iphone-se3-parametric-drawing-model (Autodesk Fusion 360 design; units mm, degrees)
part number: 2026-09-02-14-29-54-371
part number: 2026-09-02-16-09-22-957
Autodesk Fusion 360 part; units mm, degrees
sketch "スケッチ1" plane through (0, 0, 0) normal (0, 0, 1) x (1, 0, 0) in component "iPhone SE 3 - Parametric Drawing Model"
  arc A0 (33.635, 60.12) -> (24.535, 69.22) centre (24.535, 60.12) ccw
  arc A1 (24.535, -69.22) -> (33.635, -60.12) centre (24.535, -60.12) ccw
  arc A2 (-33.635, -60.12) -> (-24.535, -69.22) centre (-24.535, -60.12) ccw
  arc A3 (-24.535, 69.22) -> (-33.635, 60.12) centre (-24.535, 60.12) ccw
  line L0 (-24.535, 69.22) -> (24.535, 69.22)
  line L1 (33.635, 60.12) -> (33.635, -60.12)
  line L2 (24.535, -69.22) -> (-24.535, -69.22)
  line L3 (-33.635, -60.12) -> (-33.635, 60.12)
  dimension "d710" = 49.07
  dimension "d711" = 120.24
  dimension "d712" = 9.1
  dimension "d713" = 24.535
  dimension "d714" = 60.12
  constraint horizontal L0
  constraint horizontal L2
  constraint vertical L3
  constraint vertical L1
  constraint tangent A0 L0
  constraint tangent A0 L1
  constraint tangent A1 L1
  constraint tangent A1 L2
  constraint tangent A2 L2
  constraint tangent A2 L3
  constraint tangent A3 L3
  constraint tangent A3 L0
  constraint equal A0 A1
  constraint equal A0 A2
  constraint equal A0 A3
  measures "d710" horizontal distance of A0.end A3.start
  measures "d711" vertical distance of A0.start A1.end
  measures "d712" radius of A0
  measures "d713" horizontal distance of origin A0.centre
  measures "d714" vertical distance of origin A0.centre
extrude "Rear Glass" add sketch "スケッチ1" along normal blind 0.9 makes body 1 in component "iPhone SE 3 - Parametric Drawing Model"
ref_plane "作業平面1" through (0, 0, 0.9) normal (0, 0, 1) x (1, 0, 0) in component "iPhone SE 3 - Parametric Drawing Model"
sketch "スケッチ2" plane through (0, 0, 0.9) normal (0, 0, 1) x (1, 0, 0) in component "iPhone SE 3 - Parametric Drawing Model"
  arc A0 (33.635, 60.12) -> (24.535, 69.22) centre (24.535, 60.12) ccw
  arc A1 (24.535, -69.22) -> (33.635, -60.12) centre (24.535, -60.12) ccw
  arc A2 (-33.635, -60.12) -> (-24.535, -69.22) centre (-24.535, -60.12) ccw
  arc A3 (-24.535, 69.22) -> (-33.635, 60.12) centre (-24.535, 60.12) ccw
  line L0 (-24.535, 69.22) -> (24.535, 69.22)
  line L1 (33.635, 60.12) -> (33.635, -60.12)
  line L2 (24.535, -69.22) -> (-24.535, -69.22)
  line L3 (-33.635, -60.12) -> (-33.635, 60.12)
  dimension "d719" = 49.07
  dimension "d720" = 120.24
  dimension "d721" = 9.1
  dimension "d722" = 24.535
  dimension "d723" = 60.12
  constraint horizontal L0
  constraint horizontal L2
  constraint vertical L3
  constraint vertical L1
  constraint tangent A0 L0
  constraint tangent A0 L1
  constraint tangent A1 L1
  constraint tangent A1 L2
  constraint tangent A2 L2
  constraint tangent A2 L3
  constraint tangent A3 L3
  constraint tangent A3 L0
  constraint equal A0 A1
  constraint equal A0 A2
  constraint equal A0 A3
  measures "d719" horizontal distance of A0.end A3.start
  measures "d720" vertical distance of A0.start A1.end
  measures "d721" radius of A0
  measures "d722" horizontal distance of origin A0.centre
  measures "d723" vertical distance of origin A0.centre
extrude "Aluminum Frame" add sketch "スケッチ2" along normal blind 5.51 separate body makes body 2 in component "iPhone SE 3 - Parametric Drawing Model"
ref_plane "作業平面2" through (0, 0, 6.41) normal (0, 0, 1) x (1, 0, 0) in component "iPhone SE 3 - Parametric Drawing Model"
sketch "スケッチ3" plane through (0, 0, 6.41) normal (0, 0, 1) x (1, 0, 0) in component "iPhone SE 3 - Parametric Drawing Model"
  arc A0 (33.635, 60.12) -> (24.535, 69.22) centre (24.535, 60.12) ccw
  arc A1 (24.535, -69.22) -> (33.635, -60.12) centre (24.535, -60.12) ccw
  arc A2 (-33.635, -60.12) -> (-24.535, -69.22) centre (-24.535, -60.12) ccw
  arc A3 (-24.535, 69.22) -> (-33.635, 60.12) centre (-24.535, 60.12) ccw
  line L0 (-24.535, 69.22) -> (24.535, 69.22)
  line L1 (33.635, 60.12) -> (33.635, -60.12)
  line L2 (24.535, -69.22) -> (-24.535, -69.22)
  line L3 (-33.635, -60.12) -> (-33.635, 60.12)
  dimension "d728" = 49.07
  dimension "d729" = 120.24
  dimension "d730" = 9.1
  dimension "d731" = 24.535
  dimension "d732" = 60.12
  constraint horizontal L0
  constraint horizontal L2
  constraint vertical L3
  constraint vertical L1
  constraint tangent A0 L0
  constraint tangent A0 L1
  constraint tangent A1 L1
  constraint tangent A1 L2
  constraint tangent A2 L2
  constraint tangent A2 L3
  constraint tangent A3 L3
  constraint tangent A3 L0
  constraint equal A0 A1
  constraint equal A0 A2
  constraint equal A0 A3
  measures "d728" horizontal distance of A0.end A3.start
  measures "d729" vertical distance of A0.start A1.end
  measures "d730" radius of A0
  measures "d731" horizontal distance of origin A0.centre
  measures "d732" vertical distance of origin A0.centre
extrude "Front Cover Glass" add sketch "スケッチ3" along normal blind 0.9 separate body makes body 3 in component "iPhone SE 3 - Parametric Drawing Model"
ref_plane "作業平面3" through (0, 0, 7.31) normal (0, 0, 1) x (1, 0, 0) in component "iPhone SE 3 - Parametric Drawing Model"
sketch "スケッチ4" plane through (0, 0, 7.31) normal (0, 0, 1) x (1, 0, 0) in component "iPhone SE 3 - Parametric Drawing Model"
  arc A0 (29.25, 51.23) -> (28.45, 52.03) centre (28.45, 51.23) ccw
  arc A1 (28.45, -52.02) -> (29.25, -51.22) centre (28.45, -51.22) ccw
  arc A2 (-29.25, -51.22) -> (-28.45, -52.02) centre (-28.45, -51.22) ccw
  arc A3 (-28.45, 52.03) -> (-29.25, 51.23) centre (-28.45, 51.23) ccw
  line L0 (-28.45, 52.03) -> (28.45, 52.03)
  line L1 (29.25, 51.23) -> (29.25, -51.22)
  line L2 (28.45, -52.02) -> (-28.45, -52.02)
  line L3 (-29.25, -51.22) -> (-29.25, 51.23)
  dimension "d737" = 56.9
  dimension "d738" = 102.45
  dimension "d739" = 0.8
  dimension "d740" = 28.45
  dimension "d741" = 51.23
  constraint horizontal L0
  constraint horizontal L2
  constraint vertical L3
  constraint vertical L1
  constraint tangent A0 L0
  constraint tangent A0 L1
  constraint tangent A1 L1
  constraint tangent A1 L2
  constraint tangent A2 L2
  constraint tangent A2 L3
  constraint tangent A3 L3
  constraint tangent A3 L0
  constraint equal A0 A1
  constraint equal A0 A2
  constraint equal A0 A3
  measures "d737" horizontal distance of A0.end A3.start
  measures "d738" vertical distance of A0.start A1.end
  measures "d739" radius of A0
  measures "d740" horizontal distance of origin A0.centre
  measures "d741" vertical distance of origin A0.centre
extrude "Front Active Area Reference" add sketch "スケッチ4" along normal blind 0.02 separate body makes body 4 in component "iPhone SE 3 - Parametric Drawing Model"
sketch "スケッチ5" plane through (0, 0, 7.31) normal (0, 0, 1) x (1, 0, 0) in component "iPhone SE 3 - Parametric Drawing Model"
  circle A0 centre (0, -59.97) radius 5.45
  dimension "d744" = 59.97
  dimension "d745" = 10.9
  constraint vertical origin A0.centre
  measures "d744" vertical distance of origin A0.centre
  measures "d745" diameter of A0
extrude "Home Touch ID Sensor" add sketch "スケッチ5" along normal blind 0.02 separate body makes body 5 in component "iPhone SE 3 - Parametric Drawing Model"
sketch "スケッチ6" plane through (0, 0, 7.31) normal (0, 0, 1) x (1, 0, 0) in component "iPhone SE 3 - Parametric Drawing Model"
  circle A0 centre (-10.645, 60.12) radius 1.605
  dimension "d748" = 10.645
  dimension "d749" = 60.12
  dimension "d750" = 3.21
  measures "d748" horizontal distance of origin A0.centre
  measures "d749" vertical distance of origin A0.centre
  measures "d750" diameter of A0
extrude "Front Detail 12 Front Camera Position" add sketch "スケッチ6" along normal blind 0.02 separate body makes body 6 in component "iPhone SE 3 - Parametric Drawing Model"
sketch "スケッチ7" plane through (0, 0, 7.31) normal (0, 0, 1) x (1, 0, 0) in component "iPhone SE 3 - Parametric Drawing Model"
  circle A0 centre (-0.005, 64.38) radius 1
  dimension "d753" = 0.005
  dimension "d754" = 64.38
  dimension "d755" = 2
  measures "d753" horizontal distance of origin A0.centre
  measures "d754" vertical distance of origin A0.centre
  measures "d755" diameter of A0
extrude "Front Detail 13 Proximity Sensor Position" add sketch "スケッチ7" along normal blind 0.02 separate body makes body 7 in component "iPhone SE 3 - Parametric Drawing Model"
sketch "スケッチ8" plane through (0, 0, 7.31) normal (0, 0, 1) x (1, 0, 0) in component "iPhone SE 3 - Parametric Drawing Model"
  circle A0 centre (3.685, 64.38) radius 1
  dimension "d758" = 3.685
  dimension "d759" = 64.38
  dimension "d760" = 2
  measures "d758" horizontal distance of origin A0.centre
  measures "d759" vertical distance of origin A0.centre
  measures "d760" diameter of A0
extrude "Front Detail 14 ALS Position" add sketch "スケッチ8" along normal blind 0.02 separate body makes body 8 in component "iPhone SE 3 - Parametric Drawing Model"
sketch "スケッチ9" plane through (0, 0, 7.31) normal (0, 0, 1) x (1, 0, 0) in component "iPhone SE 3 - Parametric Drawing Model"
  arc A0 (5.335, 59.52) -> (5.335, 60.72) centre (5.335, 60.12) ccw
  arc A1 (-5.335, 60.72) -> (-5.335, 59.52) centre (-5.335, 60.12) ccw
  line L0 (-5.335, 60.72) -> (5.335, 60.72)
  line L1 (5.335, 59.52) -> (-5.335, 59.52)
  line L2 (-5.335, 60.12) -> (5.335, 60.12) construction
  point P0 (0, 60.12)
  dimension "d763" = 10.67
  dimension "d764" = 0.6
  dimension "d765" = 60.12
  constraint horizontal L0
  constraint horizontal L1
  constraint equal A0 A1
  constraint midpoint L2 P0
  constraint vertical origin P0
  measures "d763" horizontal distance of A0.centre A1.centre
  measures "d764" radius of A0
  measures "d765" vertical distance of origin P0
extrude "Receiver Opening" add sketch "スケッチ9" along normal blind 0.02 separate body makes body 9 in component "iPhone SE 3 - Parametric Drawing Model"
sketch "スケッチ10" plane through (0, 0, 0) normal (0, 0, 1) x (1, 0, 0) in component "iPhone SE 3 - Parametric Drawing Model"
  circle A0 centre (-23.195, 53.82) radius 4.285
  dimension "d768" = 23.195
  dimension "d769" = 53.82
  dimension "d770" = 8.57
  measures "d768" horizontal distance of origin A0.centre
  measures "d769" vertical distance of origin A0.centre
  measures "d770" diameter of A0
extrude "Rear Camera Bump" add sketch "スケッチ10" against normal blind 0.87 separate body makes body 10 in component "iPhone SE 3 - Parametric Drawing Model"
sketch "スケッチ11" plane through (0, 0, 0) normal (0, 0, 1) x (1, 0, 0) in component "iPhone SE 3 - Parametric Drawing Model"
  circle A0 centre (-15.505, 53.82) radius 0.75
  dimension "d773" = 15.505
  dimension "d774" = 53.82
  dimension "d775" = 1.5
  measures "d773" horizontal distance of origin A0.centre
  measures "d774" vertical distance of origin A0.centre
  measures "d775" diameter of A0
extrude "Rear Microphone" add sketch "スケッチ11" against normal blind 0.02 separate body makes body 11 in component "iPhone SE 3 - Parametric Drawing Model"
sketch "スケッチ12" plane through (0, 0, 0) normal (0, 0, 1) x (1, 0, 0) in component "iPhone SE 3 - Parametric Drawing Model"
  circle A0 centre (-10.795, 53.82) radius 1.875
  dimension "d778" = 10.795
  dimension "d779" = 53.82
  dimension "d780" = 3.75
  measures "d778" horizontal distance of origin A0.centre
  measures "d779" vertical distance of origin A0.centre
  measures "d780" diameter of A0
extrude "Rear Flash" add sketch "スケッチ12" against normal blind 0.02 separate body makes body 12 in component "iPhone SE 3 - Parametric Drawing Model"
ref_plane "作業平面4" through (-33.635, 0, 0) normal (1, 0, 0) x (0, 1, 0) in component "iPhone SE 3 - Parametric Drawing Model"
ref_plane "作業平面5" through (33.635, 0, 0) normal (1, 0, 0) x (0, 1, 0) in component "iPhone SE 3 - Parametric Drawing Model"
sketch "スケッチ13" plane through (-33.635, 0, 0) normal (1, 0, 0) x (0, 0, -1) in component "iPhone SE 3 - Parametric Drawing Model"
  arc A0 (-2.755, 50.76) -> (-4.555, 50.76) centre (-3.655, 50.76) ccw
  arc A1 (-4.555, 46.95) -> (-2.755, 46.95) centre (-3.655, 46.95) ccw
  line L0 (-2.755, 50.76) -> (-2.755, 46.95)
  line L1 (-4.555, 46.95) -> (-4.555, 50.76)
  line L2 (-3.655, 50.76) -> (-3.655, 46.95) construction
  point P0 (-3.655, 48.855)
  dimension "d787" = 3.81
  dimension "d788" = 0.9
  dimension "d789" = 3.655
  dimension "d790" = 48.855
  constraint vertical L0
  constraint vertical L1
  constraint equal A0 A1
  constraint midpoint L2 P0
  measures "d787" vertical distance of A0.centre A1.centre
  measures "d788" radius of A0
  measures "d789" horizontal distance of origin P0
  measures "d790" vertical distance of origin P0
extrude "Ring Silent Switch" add sketch "スケッチ13" against normal blind 0.42 separate body makes body 13 in component "iPhone SE 3 - Parametric Drawing Model"
sketch "スケッチ14" plane through (-33.635, 0, 0) normal (1, 0, 0) x (0, 0, -1) in component "iPhone SE 3 - Parametric Drawing Model"
  arc A0 (-2.755, 39.07) -> (-4.555, 39.07) centre (-3.655, 39.07) ccw
  arc A1 (-4.555, 30.25) -> (-2.755, 30.25) centre (-3.655, 30.25) ccw
  line L0 (-2.755, 39.07) -> (-2.755, 30.25)
  line L1 (-4.555, 30.25) -> (-4.555, 39.07)
  line L2 (-3.655, 39.07) -> (-3.655, 30.25) construction
  point P0 (-3.655, 34.66)
  dimension "d793" = 8.82
  dimension "d794" = 0.9
  dimension "d795" = 3.655
  dimension "d796" = 34.66
  constraint vertical L0
  constraint vertical L1
  constraint equal A0 A1
  constraint midpoint L2 P0
  measures "d793" vertical distance of A0.centre A1.centre
  measures "d794" radius of A0
  measures "d795" horizontal distance of origin P0
  measures "d796" vertical distance of origin P0
extrude "Volume Plus Button" add sketch "スケッチ14" against normal blind 0.4 separate body makes body 14 in component "iPhone SE 3 - Parametric Drawing Model"
sketch "スケッチ15" plane through (-33.635, 0, 0) normal (1, 0, 0) x (0, 0, -1) in component "iPhone SE 3 - Parametric Drawing Model"
  arc A0 (-2.755, 26.46) -> (-4.555, 26.46) centre (-3.655, 26.46) ccw
  arc A1 (-4.555, 17.64) -> (-2.755, 17.64) centre (-3.655, 17.64) ccw
  line L0 (-2.755, 26.46) -> (-2.755, 17.64)
  line L1 (-4.555, 17.64) -> (-4.555, 26.46)
  line L2 (-3.655, 26.46) -> (-3.655, 17.64) construction
  point P0 (-3.655, 22.05)
  dimension "d799" = 8.82
  dimension "d800" = 0.9
  dimension "d801" = 3.655
  dimension "d802" = 22.05
  constraint vertical L0
  constraint vertical L1
  constraint equal A0 A1
  constraint midpoint L2 P0
  measures "d799" vertical distance of A0.centre A1.centre
  measures "d800" radius of A0
  measures "d801" horizontal distance of origin P0
  measures "d802" vertical distance of origin P0
extrude "Volume Minus Button" add sketch "スケッチ15" against normal blind 0.4 separate body makes body 15 in component "iPhone SE 3 - Parametric Drawing Model"
sketch "スケッチ16" plane through (33.635, 0, 0) normal (1, 0, 0) x (0, 0, -1) in component "iPhone SE 3 - Parametric Drawing Model"
  arc A0 (-2.755, 38.99) -> (-4.555, 38.99) centre (-3.655, 38.99) ccw
  arc A1 (-4.555, 30.17) -> (-2.755, 30.17) centre (-3.655, 30.17) ccw
  line L0 (-2.755, 38.99) -> (-2.755, 30.17)
  line L1 (-4.555, 30.17) -> (-4.555, 38.99)
  line L2 (-3.655, 38.99) -> (-3.655, 30.17) construction
  point P0 (-3.655, 34.58)
  dimension "d805" = 8.82
  dimension "d806" = 0.9
  dimension "d807" = 3.655
  dimension "d808" = 34.58
  constraint vertical L0
  constraint vertical L1
  constraint equal A0 A1
  constraint midpoint L2 P0
  measures "d805" vertical distance of A0.centre A1.centre
  measures "d806" radius of A0
  measures "d807" horizontal distance of origin P0
  measures "d808" vertical distance of origin P0
extrude "Side Button" add sketch "スケッチ16" along normal blind 0.4 separate body makes body 16 in component "iPhone SE 3 - Parametric Drawing Model"
sketch "スケッチ17" plane through (33.635, 0, 0) normal (1, 0, 0) x (0, 0, -1) in component "iPhone SE 3 - Parametric Drawing Model"
  arc A0 (-2.505, 15.35) -> (-4.805, 15.35) centre (-3.655, 15.35) ccw
  arc A1 (-4.805, 1.98) -> (-2.505, 1.98) centre (-3.655, 1.98) ccw
  line L0 (-2.505, 15.35) -> (-2.505, 1.98)
  line L1 (-4.805, 1.98) -> (-4.805, 15.35)
  line L2 (-3.655, 15.35) -> (-3.655, 1.98) construction
  point P0 (-3.655, 8.665)
  dimension "d811" = 13.37
  dimension "d812" = 1.15
  dimension "d813" = 3.655
  dimension "d814" = 8.665
  constraint vertical L0
  constraint vertical L1
  constraint equal A0 A1
  constraint midpoint L2 P0
  measures "d811" vertical distance of A0.centre A1.centre
  measures "d812" radius of A0
  measures "d813" horizontal distance of origin P0
  measures "d814" vertical distance of origin P0
extrude "SIM Tray Seam" cut sketch "スケッチ17" against normal blind 0.05 bodies 2 in component "iPhone SE 3 - Parametric Drawing Model"
ref_plane "作業平面6" through (0, -69.22, 0) normal (0, 1, 0) x (0, 0, 1) in component "iPhone SE 3 - Parametric Drawing Model"
sketch "スケッチ18" plane through (0, -69.22, 0) normal (0, 1, 0) x (1, 0, 0) in component "iPhone SE 3 - Parametric Drawing Model"
  arc A0 (3.55, -4.455) -> (3.55, -2.855) centre (3.55, -3.655) ccw
  arc A1 (-3.55, -2.855) -> (-3.55, -4.455) centre (-3.55, -3.655) ccw
  line L0 (-3.55, -2.855) -> (3.55, -2.855)
  line L1 (3.55, -4.455) -> (-3.55, -4.455)
  line L2 (-3.55, -3.655) -> (3.55, -3.655) construction
  circle A2 centre (-23.375, -3.655) radius 0.725
  circle A3 centre (-20.975, -3.655) radius 0.725
  circle A4 centre (-18.575, -3.655) radius 0.725
  circle A5 centre (-16.175, -3.655) radius 0.725
  circle A6 centre (-13.775, -3.655) radius 0.725
  circle A7 centre (-11.375, -3.655) radius 0.725
  circle A8 centre (11.375, -3.655) radius 0.725
  circle A9 centre (13.775, -3.655) radius 0.725
  circle A10 centre (16.175, -3.655) radius 0.725
  circle A11 centre (18.575, -3.655) radius 0.725
  circle A12 centre (20.975, -3.655) radius 0.725
  circle A13 centre (23.375, -3.655) radius 0.725
  circle A14 centre (-6.395, -3.655) radius 0.8
  circle A15 centre (6.395, -3.655) radius 0.8
  point P0 (0, -3.655)
  dimension "d819" = 7.1
  dimension "d820" = 0.8
  dimension "d821" = 3.655
  dimension "d822" = 23.375
  dimension "d823" = 3.655
  dimension "d824" = 1.45
  dimension "d825" = 20.975
  dimension "d826" = 3.655
  dimension "d827" = 1.45
  dimension "d828" = 18.575
  dimension "d829" = 3.655
  dimension "d830" = 1.45
  dimension "d831" = 16.175
  dimension "d832" = 3.655
  dimension "d833" = 1.45
  dimension "d834" = 13.775
  dimension "d835" = 3.655
  dimension "d836" = 1.45
  dimension "d837" = 11.375
  dimension "d838" = 3.655
  dimension "d839" = 1.45
  dimension "d840" = 11.375
  dimension "d841" = 3.655
  dimension "d842" = 1.45
  dimension "d843" = 13.775
  dimension "d844" = 3.655
  dimension "d845" = 1.45
  dimension "d846" = 16.175
  dimension "d847" = 3.655
  dimension "d848" = 1.45
  dimension "d849" = 18.575
  dimension "d850" = 3.655
  dimension "d851" = 1.45
  dimension "d852" = 20.975
  dimension "d853" = 3.655
  dimension "d854" = 1.45
  dimension "d855" = 23.375
  dimension "d856" = 3.655
  dimension "d857" = 1.45
  dimension "d858" = 6.395
  dimension "d859" = 3.655
  dimension "d860" = 1.6
  dimension "d861" = 6.395
  dimension "d862" = 3.655
  dimension "d863" = 1.6
  constraint horizontal L0
  constraint horizontal L1
  constraint equal A0 A1
  constraint midpoint L2 P0
  constraint vertical origin P0
  measures "d819" horizontal distance of A0.centre A1.centre
  measures "d820" radius of A0
  measures "d821" vertical distance of origin P0
  measures "d822" horizontal distance of origin A2.centre
  measures "d823" vertical distance of origin A2.centre
  measures "d824" diameter of A2
  measures "d825" horizontal distance of origin A3.centre
  measures "d826" vertical distance of origin A3.centre
  measures "d827" diameter of A3
  measures "d828" horizontal distance of origin A4.centre
  measures "d829" vertical distance of origin A4.centre
  measures "d830" diameter of A4
  measures "d831" horizontal distance of origin A5.centre
  measures "d832" vertical distance of origin A5.centre
  measures "d833" diameter of A5
  measures "d834" horizontal distance of origin A6.centre
  measures "d835" vertical distance of origin A6.centre
  measures "d836" diameter of A6
  measures "d837" horizontal distance of origin A7.centre
  measures "d838" vertical distance of origin A7.centre
  measures "d839" diameter of A7
  measures "d840" horizontal distance of origin A8.centre
  measures "d841" vertical distance of origin A8.centre
  measures "d842" diameter of A8
  measures "d843" horizontal distance of origin A9.centre
  measures "d844" vertical distance of origin A9.centre
  measures "d845" diameter of A9
  measures "d846" horizontal distance of origin A10.centre
  measures "d847" vertical distance of origin A10.centre
  measures "d848" diameter of A10
  measures "d849" horizontal distance of origin A11.centre
  measures "d850" vertical distance of origin A11.centre
  measures "d851" diameter of A11
  measures "d852" horizontal distance of origin A12.centre
  measures "d853" vertical distance of origin A12.centre
  measures "d854" diameter of A12
  measures "d855" horizontal distance of origin A13.centre
  measures "d856" vertical distance of origin A13.centre
  measures "d857" diameter of A13
  measures "d858" horizontal distance of origin A14.centre
  measures "d859" vertical distance of origin A14.centre
  measures "d860" diameter of A14
  measures "d861" horizontal distance of origin A15.centre
  measures "d862" vertical distance of origin A15.centre
  measures "d863" diameter of A15
extrude "Bottom Port and Acoustic Openings" cut sketch "スケッチ18" along normal blind 1 bodies 2 in component "iPhone SE 3 - Parametric Drawing Model"
ref_plane "作業平面7" through (0, 0, 3.655) normal (0, 0, 1) x (1, 0, 0) in component "iPhone SE 3 - Parametric Drawing Model"
sketch "スケッチ19" plane through (0, 0, 3.655) normal (0, 0, 1) x (1, 0, 0) in component "iPhone SE 3 - Parametric Drawing Model"
  arc A0 (33.635, 60.12) -> (24.535, 69.22) centre (24.535, 60.12) ccw
  arc A1 (24.535, -69.22) -> (33.635, -60.12) centre (24.535, -60.12) ccw
  arc A2 (-33.635, -60.12) -> (-24.535, -69.22) centre (-24.535, -60.12) ccw
  arc A3 (-24.535, 69.22) -> (-33.635, 60.12) centre (-24.535, 60.12) ccw
  line L0 (-24.535, 69.22) -> (24.535, 69.22)
  line L1 (33.635, 60.12) -> (33.635, -60.12)
  line L2 (24.535, -69.22) -> (-24.535, -69.22)
  line L3 (-33.635, -60.12) -> (-33.635, 60.12)
  dimension "d868" = 49.07
  dimension "d869" = 120.24
  dimension "d870" = 9.1
  dimension "d871" = 24.535
  dimension "d872" = 60.12
  constraint horizontal L0
  constraint horizontal L2
  constraint vertical L3
  constraint vertical L1
  constraint tangent A0 L0
  constraint tangent A0 L1
  constraint tangent A1 L1
  constraint tangent A1 L2
  constraint tangent A2 L2
  constraint tangent A2 L3
  constraint tangent A3 L3
  constraint tangent A3 L0
  constraint equal A0 A1
  constraint equal A0 A2
  constraint equal A0 A3
  measures "d868" horizontal distance of A0.end A3.start
  measures "d869" vertical distance of A0.start A1.end
  measures "d870" radius of A0
  measures "d871" horizontal distance of origin A0.centre
  measures "d872" vertical distance of origin A0.centre
component "iPhone SE 3 - Parametric Drawing Model" placed x (1, 0, 0) y (0, 1, 0) z (0, 0, 1) at (0, 0, 0)
equation "SE3_OverallWidth = 67.27 mm" comment "Overall product width"
equation "SE3_OverallHeight = 138.44 mm" comment "Overall product height"
equation "SE3_ProductThickness = 7.31 mm" comment "Nominal product thickness"
equation "SE3_CornerRadius = 9.10 mm" comment "Parameterized plan-view corner radius"
equation "SE3_RearGlassThickness = 0.90 mm" comment "Modeled rear glass thickness"
equation "SE3_FrontGlassThickness = 0.90 mm" comment "Modeled front glass thickness"
equation "SE3_ActiveWidth = 58.50 mm" comment "Front active-area width"
equation "SE3_ActiveHeight = 104.05 mm" comment "Front active-area height"
equation "SE3_ActiveTopOffset = 17.19 mm" comment "Top product datum to active area"
equation "SE3_HomeDiameter = 10.90 mm" comment "Home/Touch ID sensor diameter"
equation "SE3_HomeBottomOffset = 9.25 mm" comment "Bottom datum to Home sensor center"
equation "SE3_ReceiverWidth = 11.87 mm" comment "Receiver width"
equation "SE3_ReceiverHeight = 1.20 mm" comment "Receiver height"
equation "SE3_ReceiverTopOffset = 9.10 mm" comment "Top datum to receiver center"
equation "SE3_FrontCameraDiameter = 3.21 mm" comment "Front camera opening/keepout diameter"
equation "SE3_FrontCameraXFromLeft = 22.99 mm" comment "Left datum to front camera center"
equation "SE3_FrontCameraTopOffset = 9.10 mm" comment "Top datum to front camera center"
equation "SE3_ProximityDiameter = 2.00 mm" comment "Proximity sensor display diameter"
equation "SE3_ProximityXFromLeft = 33.63 mm" comment "Left datum to proximity center"
equation "SE3_ProximityTopOffset = 4.84 mm" comment "Top datum to proximity center"
equation "SE3_ALSDiameter = 2.00 mm" comment "Ambient light sensor display diameter"
equation "SE3_ALSXFromLeft = 37.32 mm" comment "Left datum to ALS center"
equation "SE3_ALSTopOffset = 4.84 mm" comment "Top datum to ALS center"
equation "SE3_RearCameraDiameter = 8.57 mm" comment "Rear camera opening diameter"
equation "SE3_RearMicDiameter = 1.50 mm" comment "Rear microphone diameter"
equation "SE3_RearFlashDiameter = 3.75 mm" comment "Rear flash diameter"
equation "SE3_RearCameraXFromLeft = 10.44 mm" comment "Left datum to rear camera center"
equation "SE3_RearMicXFromLeft = 18.13 mm" comment "Left datum to rear microphone center"
equation "SE3_RearFlashXFromLeft = 22.84 mm" comment "Left datum to rear flash center"
equation "SE3_RearFeatureTopOffset = 15.40 mm" comment "Top datum to rear feature centers"
equation "SE3_CameraBumpHeight = 0.87 mm" comment "Modeled rear camera projection"
equation "SE3_RingTopOffset = 17.56 mm" comment "Top datum to top of ring/silent switch"
equation "SE3_RingLength = 5.61 mm" comment "Ring/silent switch length"
equation "SE3_VolumePlusCenterFromTop = 34.56 mm" comment "Top datum to volume-plus center"
equation "SE3_VolumeMinusCenterFromTop = 47.17 mm" comment "Top datum to volume-minus center"
equation "SE3_ButtonLength = 10.62 mm" comment "Button length: 2 x 5.31"
equation "SE3_ButtonFaceWidth = 1.80 mm" comment "Modeled button width in product-thickness direction"
equation "SE3_RingProjection = 0.42 mm" comment "Ring/silent switch projection"
equation "SE3_ButtonProjection = 0.40 mm" comment "Volume and side-button projection"
equation "SE3_SideButtonCenterFromTop = 34.64 mm" comment "Top datum to side-button center"
equation "SE3_SIMTrayTopOffset = 52.72 mm" comment "Top datum to SIM tray top"
equation "SE3_SIMTrayLength = 15.67 mm" comment "SIM tray length"
equation "SE3_SIMTrayWidth = 2.30 mm" comment "SIM tray visible width"
equation "SE3_BottomHoleDiameter = 1.45 mm" comment "Bottom microphone/speaker hole diameter"
equation "SE3_BottomHoleFirstFromLeft = 10.26 mm" comment "Left datum to first left acoustic hole"
equation "SE3_BottomHolePitch = 2.40 mm" comment "Bottom acoustic-hole pitch: 12.00 / 5"
equation "SE3_BottomRightFirstFromLeft = 45.01 mm" comment "Left datum to first right acoustic hole"
equation "SE3_ScrewDiameter = 1.60 mm" comment "Bottom screw diameter"
equation "SE3_LeftScrewFromLeft = 27.24 mm" comment "Left datum to left screw"
equation "SE3_RightScrewFromLeft = 40.03 mm" comment "Left datum to right screw"
equation "SE3_LightningWidth = 8.70 mm" comment "Lightning opening width: 37.98 - 29.28"
equation "SE3_LightningHeight = 1.60 mm" comment "Modeled Lightning opening height"
equation "SE3_DetailOverlay = 0.02 mm" comment "Visual reference overlay thickness"
equation "d710 = SE3_OverallWidth - 2 * SE3_CornerRadius"
equation "d711 = SE3_OverallHeight - 2 * SE3_CornerRadius"
equation "d712 = SE3_CornerRadius"
equation "d713 = SE3_OverallWidth / 2 - SE3_CornerRadius"
equation "d714 = SE3_OverallHeight / 2 - SE3_CornerRadius"
equation "d715 = SE3_RearGlassThickness"
equation "d717 = SE3_RearGlassThickness"
equation "d719 = SE3_OverallWidth - 2 * SE3_CornerRadius"
equation "d720 = SE3_OverallHeight - 2 * SE3_CornerRadius"
equation "d721 = SE3_CornerRadius"
equation "d722 = SE3_OverallWidth / 2 - SE3_CornerRadius"
equation "d723 = SE3_OverallHeight / 2 - SE3_CornerRadius"
equation "d724 = SE3_ProductThickness - SE3_RearGlassThickness - SE3_FrontGlassThickness"
equation "d726 = SE3_ProductThickness - SE3_FrontGlassThickness"
equation "d728 = SE3_OverallWidth - 2 * SE3_CornerRadius"
equation "d729 = SE3_OverallHeight - 2 * SE3_CornerRadius"
equation "d730 = SE3_CornerRadius"
equation "d731 = SE3_OverallWidth / 2 - SE3_CornerRadius"
equation "d732 = SE3_OverallHeight / 2 - SE3_CornerRadius"
equation "d733 = SE3_FrontGlassThickness"
equation "d735 = SE3_ProductThickness"
equation "d737 = SE3_ActiveWidth - 2 * 0.80 mm"
equation "d738 = SE3_ActiveHeight - 2 * 0.80 mm"
equation "d740 = SE3_ActiveWidth / 2 - 0.80 mm"
equation "d741 = ( SE3_OverallHeight / 2 - SE3_ActiveTopOffset - SE3_ActiveHeight / 2 ) + SE3_ActiveHeight / 2 - 0.80 mm"
equation "d742 = SE3_DetailOverlay"
equation "d744 = SE3_OverallHeight / 2 - SE3_HomeBottomOffset"
equation "d745 = SE3_HomeDiameter"
equation "d746 = SE3_DetailOverlay"
equation "d748 = SE3_OverallWidth / 2 - SE3_FrontCameraXFromLeft"
equation "d749 = SE3_OverallHeight / 2 - SE3_FrontCameraTopOffset"
equation "d750 = SE3_FrontCameraDiameter"
equation "d751 = SE3_DetailOverlay"
equation "d753 = SE3_OverallWidth / 2 - SE3_ProximityXFromLeft"
equation "d754 = SE3_OverallHeight / 2 - SE3_ProximityTopOffset"
equation "d755 = SE3_ProximityDiameter"
equation "d756 = SE3_DetailOverlay"
equation "d758 = SE3_ALSXFromLeft - SE3_OverallWidth / 2"
equation "d759 = SE3_OverallHeight / 2 - SE3_ALSTopOffset"
equation "d760 = SE3_ALSDiameter"
equation "d761 = SE3_DetailOverlay"
equation "d763 = SE3_ReceiverWidth - SE3_ReceiverHeight"
equation "d764 = SE3_ReceiverHeight / 2"
equation "d765 = SE3_OverallHeight / 2 - SE3_ReceiverTopOffset"
equation "d766 = SE3_DetailOverlay"
equation "d768 = SE3_OverallWidth / 2 - SE3_RearCameraXFromLeft"
equation "d769 = SE3_OverallHeight / 2 - SE3_RearFeatureTopOffset"
equation "d770 = SE3_RearCameraDiameter"
equation "d771 = -( SE3_CameraBumpHeight )"
equation "d773 = SE3_OverallWidth / 2 - SE3_RearMicXFromLeft"
equation "d774 = SE3_OverallHeight / 2 - SE3_RearFeatureTopOffset"
equation "d775 = SE3_RearMicDiameter"
equation "d776 = -( SE3_DetailOverlay )"
equation "d778 = SE3_OverallWidth / 2 - SE3_RearFlashXFromLeft"
equation "d779 = SE3_OverallHeight / 2 - SE3_RearFeatureTopOffset"
equation "d780 = SE3_RearFlashDiameter"
equation "d781 = -( SE3_DetailOverlay )"
equation "d783 = -SE3_OverallWidth / 2"
equation "d785 = SE3_OverallWidth / 2"
equation "d787 = SE3_RingLength - SE3_ButtonFaceWidth"
equation "d788 = SE3_ButtonFaceWidth / 2"
equation "d789 = SE3_ProductThickness / 2"
equation "d790 = SE3_OverallHeight / 2 - SE3_RingTopOffset - SE3_RingLength / 2"
equation "d791 = -( SE3_RingProjection )"
equation "d793 = SE3_ButtonLength - SE3_ButtonFaceWidth"
equation "d794 = SE3_ButtonFaceWidth / 2"
equation "d795 = SE3_ProductThickness / 2"
equation "d796 = SE3_OverallHeight / 2 - SE3_VolumePlusCenterFromTop"
equation "d797 = -( SE3_ButtonProjection )"
equation "d799 = SE3_ButtonLength - SE3_ButtonFaceWidth"
equation "d800 = SE3_ButtonFaceWidth / 2"
equation "d801 = SE3_ProductThickness / 2"
equation "d802 = SE3_OverallHeight / 2 - SE3_VolumeMinusCenterFromTop"
equation "d803 = -( SE3_ButtonProjection )"
equation "d805 = SE3_ButtonLength - SE3_ButtonFaceWidth"
equation "d806 = SE3_ButtonFaceWidth / 2"
equation "d807 = SE3_ProductThickness / 2"
equation "d808 = SE3_OverallHeight / 2 - SE3_SideButtonCenterFromTop"
equation "d809 = SE3_ButtonProjection"
equation "d811 = SE3_SIMTrayLength - SE3_SIMTrayWidth"
equation "d812 = SE3_SIMTrayWidth / 2"
equation "d813 = SE3_ProductThickness / 2"
equation "d814 = SE3_OverallHeight / 2 - SE3_SIMTrayTopOffset - SE3_SIMTrayLength / 2"
equation "d815 = -( 0.05 mm )"
equation "d817 = -SE3_OverallHeight / 2"
equation "d819 = SE3_LightningWidth - SE3_LightningHeight"
equation "d820 = SE3_LightningHeight / 2"
equation "d821 = SE3_ProductThickness / 2"
equation "d822 = SE3_OverallWidth / 2 - ( SE3_BottomHoleFirstFromLeft + 0 * SE3_BottomHolePitch )"
equation "d823 = SE3_ProductThickness / 2"
equation "d824 = SE3_BottomHoleDiameter"
equation "d825 = SE3_OverallWidth / 2 - ( SE3_BottomHoleFirstFromLeft + 1 * SE3_BottomHolePitch )"
equation "d826 = SE3_ProductThickness / 2"
equation "d827 = SE3_BottomHoleDiameter"
equation "d828 = SE3_OverallWidth / 2 - ( SE3_BottomHoleFirstFromLeft + 2 * SE3_BottomHolePitch )"
equation "d829 = SE3_ProductThickness / 2"
equation "d830 = SE3_BottomHoleDiameter"
equation "d831 = SE3_OverallWidth / 2 - ( SE3_BottomHoleFirstFromLeft + 3 * SE3_BottomHolePitch )"
equation "d832 = SE3_ProductThickness / 2"
equation "d833 = SE3_BottomHoleDiameter"
equation "d834 = SE3_OverallWidth / 2 - ( SE3_BottomHoleFirstFromLeft + 4 * SE3_BottomHolePitch )"
equation "d835 = SE3_ProductThickness / 2"
equation "d836 = SE3_BottomHoleDiameter"
equation "d837 = SE3_OverallWidth / 2 - ( SE3_BottomHoleFirstFromLeft + 5 * SE3_BottomHolePitch )"
equation "d838 = SE3_ProductThickness / 2"
equation "d839 = SE3_BottomHoleDiameter"
equation "d840 = ( SE3_BottomRightFirstFromLeft + 0 * SE3_BottomHolePitch ) - SE3_OverallWidth / 2"
equation "d841 = SE3_ProductThickness / 2"
equation "d842 = SE3_BottomHoleDiameter"
equation "d843 = ( SE3_BottomRightFirstFromLeft + 1 * SE3_BottomHolePitch ) - SE3_OverallWidth / 2"
equation "d844 = SE3_ProductThickness / 2"
equation "d845 = SE3_BottomHoleDiameter"
equation "d846 = ( SE3_BottomRightFirstFromLeft + 2 * SE3_BottomHolePitch ) - SE3_OverallWidth / 2"
equation "d847 = SE3_ProductThickness / 2"
equation "d848 = SE3_BottomHoleDiameter"
equation "d849 = ( SE3_BottomRightFirstFromLeft + 3 * SE3_BottomHolePitch ) - SE3_OverallWidth / 2"
equation "d850 = SE3_ProductThickness / 2"
equation "d851 = SE3_BottomHoleDiameter"
equation "d852 = ( SE3_BottomRightFirstFromLeft + 4 * SE3_BottomHolePitch ) - SE3_OverallWidth / 2"
equation "d853 = SE3_ProductThickness / 2"
equation "d854 = SE3_BottomHoleDiameter"
equation "d855 = ( SE3_BottomRightFirstFromLeft + 5 * SE3_BottomHolePitch ) - SE3_OverallWidth / 2"
equation "d856 = SE3_ProductThickness / 2"
equation "d857 = SE3_BottomHoleDiameter"
equation "d858 = SE3_OverallWidth / 2 - SE3_LeftScrewFromLeft"
equation "d859 = SE3_ProductThickness / 2"
equation "d860 = SE3_ScrewDiameter"
equation "d861 = SE3_RightScrewFromLeft - SE3_OverallWidth / 2"
equation "d862 = SE3_ProductThickness / 2"
equation "d863 = SE3_ScrewDiameter"
equation "d866 = SE3_ProductThickness / 2"
equation "d868 = SE3_OverallWidth - 2 * SE3_CornerRadius"
equation "d869 = SE3_OverallHeight - 2 * SE3_CornerRadius"
equation "d870 = SE3_CornerRadius"
equation "d871 = SE3_OverallWidth / 2 - SE3_CornerRadius"
equation "d872 = SE3_OverallHeight / 2 - SE3_CornerRadius"
named bodies: "Rear Glass", "Aluminum Frame", "Front Cover Glass", "Front Active Area Reference", "Home Touch ID Sensor", "Front Detail 12 Front Camera Position", "Front Detail 13 Proximity Sensor Position", "Front Detail 14 ALS Position", "Receiver Opening", "Rear Camera Bump", "Rear Microphone", "Rear Flash", "Ring Silent Switch", "Volume Plus Button", "Volume Minus Button", "Side Button"
